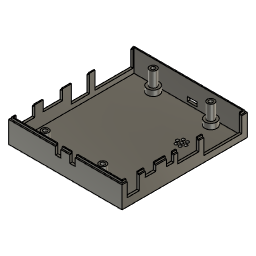
VersaTermTop (Autodesk Fusion 360 design; units mm, degrees)
Autodesk Fusion 360 part; units mm, degrees
(part 1 of 3)
box "BoxPrimitive1" add length 104.5 width 94.5 height 20.6 placed x (0, 1, 0) y (-1, 0, 0) z (0, 0, 1) at (94.5, 0, 0) makes body 1
shell "Shell1" thickness 2 removed faces 1 at (31.5, 34.8333, 20.6) on bodies 1
sketch "Sketch3" plane through (0, 0, 2) normal (0, 0, 1) x (-1, 0, 0)
  line L0 (-92.5, -102.5) -> (-2, -102.5)
  line L1 (-2, -102.5) -> (-2, -2)
  line L2 (-2, -2) -> (-92.5, -2)
  line L3 (-92.5, -2) -> (-92.5, -102.5)
  circle A0 centre (-23.25, -97.25) radius 5
  dimension "d7" = 10
  dimension "d8" = 5.25
  dimension "d9" = 21.25
  measures "d7" diameter of A0
  measures "d8" distance of L0 A0.centre
  measures "d9" distance of L1 A0.centre
extrude "Extrude1" add sketch "Sketch3" along normal blind 4.6 contours A0 bodies 1
sketch "Sketch16" plane through (0, 0, 6.6) normal (0, 0, 1) x (-1, 0, 0)
  circle A0 centre (-23.25, -97.25) radius 5
  circle A1 centre (-23.25, -97.25) radius 3
  dimension "d42" = 6
  constraint concentric A0 A1
  measures "d42" diameter of A1
extrude "Extrude7" add sketch "Sketch16" along normal blind 12.4 contours A1 bodies 1
sketch "Sketch18" plane through (0, 0, 2) normal (0, 0, 1) x (-1, 0, 0)
  circle A0 centre (-23.25, -97.25) radius 5
  line L0 (-92.5, -102.5) -> (-2, -102.5)
  line L1 (-2, -102.5) -> (-2, -2)
  line L2 (-2, -2) -> (-92.5, -2)
  line L3 (-92.5, -2) -> (-92.5, -102.5)
  circle A1 centre (-23.25, -97.25) radius 3.125
  dimension "d49" = 6.25
  constraint concentric A0 A1
  measures "d49" diameter of A1
extrude "Extrude8" cut sketch "Sketch18" against normal blind 3.1 from surface at 1.1 contours A1 bodies 1
sketch "Sketch20" plane through (0, 0, 3.1) normal (0, 0, -1) x (1, 0, 0)
  circle A0 centre (23.25, -97.25) radius 3.125
  circle A1 centre (23.25, -97.25) radius 1.65
  dimension "d56" = 3.3
  constraint concentric A0 A1
  measures "d56" diameter of A1
extrude "Extrude10" cut sketch "Sketch20" against normal blind 17 contours A1 bodies 1
pattern_linear "R-Pattern3" count 2 spacing 90 along (0, -1, 0) count 2 spacing 48 along (1, 0, 0) of "Extrude1", "Extrude7", "Extrude8", "Extrude10"
chamfer "Chamfer2" distance 1 angle 45 4 edges at (94.5, 52.25, 0) (47.25, 0, 0) (47.25, 104.5, 0) (0, 52.25, 0) on bodies 1
sketch "Sketch39" plane through (0, 0, 20.6) normal (0, 0, 1) x (-1, 0, 0)
  line L0 (-92.5, -102.5) -> (-92.5, -2)
  line L1 (-92.5, -2) -> (-2, -2)
  line L2 (-2, -2) -> (-2, -102.5)
  line L3 (-2, -102.5) -> (-92.5, -102.5)
  line L4 (-94.5, -104.5) -> (0, -104.5)
  line L5 (0, -104.5) -> (0, 0)
  line L6 (0, 0) -> (-94.5, 0)
  line L7 (-94.5, 0) -> (-94.5, -104.5)
  line L8 (0, -104.5) -> (-94.5, -104.5)
  line L9 (-94.5, -104.5) -> (-94.5, 0)
  line L10 (-94.5, 0) -> (0, 0)
  line L11 (0, 0) -> (0, -104.5)
  line L12 (-93.4, -1.1) -> (-1.1, -1.1)
  line L13 (-1.1, -1.1) -> (-1.1, -103.4)
  line L14 (-1.1, -103.4) -> (-93.4, -103.4)
  line L15 (-93.4, -103.4) -> (-93.4, -1.1)
  dimension "d89" = 1.1
  constraint horizontal L8
  constraint vertical L9
  constraint horizontal L10
  constraint vertical L11
  constraint coincident L6.end L7.start
  constraint coincident L4.end L5.start
extrude "Extrude15" cut sketch "Sketch39" against normal blind 1.6 contours L4 L5 L6 L7 L8 L9 L10 L11 bodies 1
sketch "Sketch27" plane through (94.5, 0, 0) normal (1, 0, 0) x (0, 1, 0)
  line L0 (104.5, 1) -> (104.5, 19)
  line L1 (0, 19) -> (0, 1)
  line L2 (4.39, 20.6) -> (14.39, 20.6)
  line L3 (14.39, 20.6) -> (14.39, 7.6)
  line L4 (14.39, 7.6) -> (4.39, 7.6)
  line L5 (4.39, 7.6) -> (4.39, 20.6)
  line L6 (0, 1) -> (104.5, 1)
  line L7 (104.5, 19) -> (0, 19)
  line L8 (1.1, 20.6) -> (103.4, 20.6)
  dimension "d69" = 13
  dimension "d70" = 10
  dimension "d79" = 4.39
  constraint horizontal L2
  constraint vertical L3
  constraint horizontal L4
  constraint vertical L5
  constraint collinear L2 L8
  measures "d69" distance of L2 L4
  measures "d70" distance of L3 L5
  measures "d79" distance of L1 L5
extrude "Extrude12" cut sketch "Sketch27" against normal blind 2 contours L2 L3 L5 L7 L8 | L3 L4 L5 L7 bodies 1
sketch "Sketch28" plane through (94.5, 0, 0) normal (1, 0, 0) x (0, 1, 0)
  line L0 (0, 19) -> (0, 1)
  line L1 (104.5, 1) -> (104.5, 19)
  line L2 (19.465, 20.6) -> (28.165, 20.6)
  line L3 (28.165, 20.6) -> (28.165, 14.7)
  line L4 (28.165, 14.7) -> (19.465, 14.7)
  line L5 (19.465, 14.7) -> (19.465, 20.6)
  line L6 (4.39, 7.6) -> (4.39, 19)
  line L7 (14.39, 19) -> (14.39, 7.6)
  line L8 (14.39, 7.6) -> (4.39, 7.6)
  line L9 (0, 1) -> (104.5, 1)
  line L10 (4.39, 19) -> (0, 19)
  line L11 (104.5, 19) -> (14.39, 19)
  line L12 (14.39, 20.6) -> (103.4, 20.6)
  dimension "d75" = 8.7
  dimension "d76" = 5.9
  dimension "d80" = 19.465
  constraint horizontal L2
  constraint vertical L3
  constraint horizontal L4
  constraint vertical L5
  constraint collinear L2 L12
  measures "d75" distance of L3 L5
  measures "d76" distance of L2 L4
  measures "d80" distance of L0 L5
extrude "Extrude13" cut sketch "Sketch28" against normal blind 2 contours L2 L3 L5 L11 L12 | L3 L4 L5 L11 bodies 1
sketch "Sketch41" plane through (0, 0, 0) normal (-1, 0, 0) x (0, -1, 0)
  line L0 (-104.5, 19) -> (-104.5, 1)
  line L1 (0, 1) -> (0, 19)
  line L2 (-65.35, 20.6) -> (-50.35, 20.6)
  line L3 (-50.35, 20.6) -> (-50.35, 5.8)
  line L4 (-50.35, 5.8) -> (-65.35, 5.8)
  line L5 (-65.35, 5.8) -> (-65.35, 20.6)
  line L6 (-104.5, 1) -> (0, 1)
  line L7 (0, 19) -> (-104.5, 19)
  line L8 (-28.165, 20.6) -> (-103.4, 20.6)
  dimension "d97" = 14.8
  dimension "d98" = 15
  dimension "d102" = 39.15
  constraint horizontal L2
  constraint vertical L3
  constraint horizontal L4
  constraint vertical L5
  constraint collinear L2 L8
  measures "d97" distance of L2 L4
  measures "d98" distance of L3 L5
  measures "d102" distance of L0 L5
extrude "Extrude17" cut sketch "Sketch41" against normal blind 2 contours L3 L4 L5 L7 | L2 L3 L5 L7 L8 bodies 1
sketch "Sketch42" plane through (0, 0, 0) normal (-1, 0, 0) x (0, -1, 0)
  line L0 (-65.35, 5.8) -> (-65.35, 19)
  line L1 (-104.5, 19) -> (-104.5, 1)
  line L2 (0, 1) -> (0, 19)
  line L3 (-50.35, 19) -> (-50.35, 5.8)
  line L4 (-50.35, 5.8) -> (-65.35, 5.8)
  line L5 (-42.94, 20.6) -> (-26.94, 20.6)
  line L6 (-26.94, 20.6) -> (-26.94, 12)
  line L7 (-26.94, 12) -> (-42.94, 12)
  line L8 (-42.94, 12) -> (-42.94, 20.6)
  line L9 (-104.5, 1) -> (0, 1)
  line L10 (-65.35, 19) -> (-104.5, 19)
  line L11 (0, 19) -> (-50.35, 19)
  line L12 (-28.165, 20.6) -> (-103.4, 20.6)
  dimension "d103" = 16
  dimension "d104" = 8.6
  dimension "d105" = 26.94
  constraint horizontal L5
  constraint vertical L6
  constraint horizontal L7
  constraint vertical L8
  constraint collinear L5 L12
  measures "d103" distance of L6 L8
  measures "d104" distance of L5 L7
  measures "d105" distance of L2 L6
extrude "Extrude18" cut sketch "Sketch42" against normal blind 2 contours L6 L7 L8 L11 | L5 L6 L8 L11 L12 bodies 1
sketch "Sketch43" plane through (0, 0, 0) normal (-1, 0, 0) x (0, -1, 0)
  line L0 (-42.94, 12) -> (-42.94, 19)
  line L1 (-50.35, 19) -> (-50.35, 5.8)
  line L2 (-50.35, 5.8) -> (-65.35, 5.8)
  line L3 (-65.35, 5.8) -> (-65.35, 19)
  line L4 (-104.5, 19) -> (-104.5, 1)
  line L5 (0, 1) -> (0, 19)
  line L6 (-26.94, 19) -> (-26.94, 12)
  line L7 (-26.94, 12) -> (-42.94, 12)
  line L8 (-19.83, 20.6) -> (-4.33, 20.6)
  line L9 (-4.33, 20.6) -> (-4.33, 11.5)
  line L10 (-4.33, 11.5) -> (-19.83, 11.5)
  line L11 (-19.83, 11.5) -> (-19.83, 20.6)
  line L12 (-104.5, 1) -> (0, 1)
  line L13 (-42.94, 19) -> (-50.35, 19)
  line L14 (-65.35, 19) -> (-104.5, 19)
  line L15 (0, 19) -> (-26.94, 19)
  line L16 (-2, 20.6) -> (-26.94, 20.6)
  dimension "d108" = 4.33
  dimension "d109" = 15.5
  dimension "d110" = 9.1
  constraint horizontal L8
  constraint vertical L9
  constraint horizontal L10
  constraint vertical L11
  constraint collinear L8 L16
  measures "d108" distance of L5 L9
  measures "d109" distance of L9 L11
  measures "d110" distance of L8 L10
extrude "Extrude19" cut sketch "Sketch43" against normal blind 2 contours L9 L10 L11 L15 | L8 L9 L11 L15 L16 bodies 1
sketch "Sketch44" plane through (0, 0, 0) normal (-1, 0, 0) x (0, -1, 0)
  line L0 (-19.83, 11.5) -> (-19.83, 19)
  line L1 (-26.94, 19) -> (-26.94, 12)
  line L2 (-26.94, 12) -> (-42.94, 12)
  line L3 (-42.94, 12) -> (-42.94, 19)
  line L4 (-50.35, 19) -> (-50.35, 5.8)
  line L5 (-50.35, 5.8) -> (-65.35, 5.8)
  line L6 (-65.35, 5.8) -> (-65.35, 19)
  line L7 (-104.5, 19) -> (-104.5, 1)
  line L8 (0, 1) -> (0, 19)
  line L9 (-4.33, 19) -> (-4.33, 11.5)
  line L10 (-4.33, 11.5) -> (-19.83, 11.5)
  line L11 (-101.776, 20.6) -> (-69.966, 20.6)
  line L12 (-69.966, 20.6) -> (-69.966, 6.05)
  line L13 (-69.966, 6.05) -> (-101.776, 6.05)
  line L14 (-101.776, 6.05) -> (-101.776, 20.6)
  line L15 (-104.5, 1) -> (0, 1)
  line L16 (-19.83, 19) -> (-26.94, 19)
  line L17 (-42.94, 19) -> (-50.35, 19)
  line L18 (-65.35, 19) -> (-104.5, 19)
  line L19 (0, 19) -> (-4.33, 19)
  line L20 (-28.165, 20.6) -> (-103.4, 20.6)
  dimension "d113" = 31.81
  dimension "d114" = 14.55
  dimension "d115" = 2.724
  constraint horizontal L11
  constraint vertical L12
  constraint horizontal L13
  constraint vertical L14
  constraint collinear L11 L20
  measures "d113" distance of L12 L14
  measures "d114" distance of L11 L13
  measures "d115" distance of L7 L14
extrude "Extrude20" cut sketch "Sketch44" against normal blind 2 contours L12 L13 L14 L18 | L11 L12 L14 L18 L20 bodies 1
sketch "Sketch45" plane through (94.5, 0, 0) normal (1, 0, 0) x (0, 1, 0)
  line L0 (46.5, 20.6) -> (64, 20.6)
  line L1 (64, 20.6) -> (64, 10.9)
  line L2 (64, 10.9) -> (46.5, 10.9)
  line L3 (46.5, 10.9) -> (46.5, 20.6)
  line L4 (104.5, 1) -> (104.5, 18.5)
  line L5 (19.465, 14.7) -> (19.465, 19)
  line L6 (14.39, 19) -> (14.39, 7.6)
  line L7 (14.39, 7.6) -> (4.39, 7.6)
  line L8 (4.39, 7.6) -> (4.39, 19)
  line L9 (0, 19) -> (0, 1)
  line L10 (0, 1) -> (104.5, 1)
  line L11 (104.5, 1) -> (104.5, 19)
  line L12 (28.165, 19) -> (28.165, 14.7)
  line L13 (28.165, 14.7) -> (19.465, 14.7)
  line L14 (19.465, 19) -> (14.39, 19)
  line L15 (4.39, 19) -> (0, 19)
  line L16 (104.5, 19) -> (28.165, 19)
  line L17 (28.165, 20.6) -> (103.4, 20.6)
  dimension "d118" = 40.5
  dimension "d119" = 17.5
  dimension "d120" = 9.7
  constraint horizontal L0
  constraint vertical L1
  constraint horizontal L2
  constraint vertical L3
  constraint collinear L0 L17
  measures "d118" distance of L1 L4
  measures "d119" distance of L1 L3
  measures "d120" distance of L0 L2
extrude "Extrude21" cut sketch "Sketch45" against normal blind 2 contours L0 L1 L3 L16 L17 | L1 L2 L3 L16 bodies 1
sketch "Sketch46" plane through (94.5, 0, 0) normal (1, 0, 0) x (0, 1, 0)
  line L0 (46.5, 10.9) -> (46.5, 19)
  line L1 (28.165, 19) -> (28.165, 14.7)
  line L2 (28.165, 14.7) -> (19.465, 14.7)
  line L3 (19.465, 14.7) -> (19.465, 19)
  line L4 (14.39, 19) -> (14.39, 7.6)
  line L5 (14.39, 7.6) -> (4.39, 7.6)
  line L6 (4.39, 7.6) -> (4.39, 19)
  line L7 (0, 19) -> (0, 1)
  line L8 (0, 1) -> (104.5, 1)
  line L9 (104.5, 1) -> (104.5, 19)
  line L10 (64, 19) -> (64, 10.9)
  line L11 (64, 10.9) -> (46.5, 10.9)
  line L12 (68.186, 20.6) -> (99.746, 20.6)
  line L13 (99.746, 20.6) -> (99.746, 6.05)
  line L14 (99.746, 6.05) -> (68.186, 6.05)
  line L15 (68.186, 6.05) -> (68.186, 20.6)
  line L16 (46.5, 19) -> (28.165, 19)
  line L17 (19.465, 19) -> (14.39, 19)
  line L18 (4.39, 19) -> (0, 19)
  line L19 (104.5, 19) -> (64, 19)
  line L20 (64, 20.6) -> (103.4, 20.6)
  dimension "d124" = 4.754
  dimension "d125" = 31.56
  dimension "d126" = 14.55
  constraint horizontal L12
  constraint vertical L13
  constraint horizontal L14
  constraint vertical L15
  constraint collinear L12 L20
  measures "d124" distance of L9 L13
  measures "d125" distance of L13 L15
  measures "d126" distance of L12 L14
extrude "Extrude22" cut sketch "Sketch46" against normal blind 2 contours L13 L14 L15 L19 | L12 L13 L15 L19 L20 bodies 1
sketch "Sketch47" plane through (94.5, 0, 0) normal (1, 0, 0) x (0, 1, 0)
  line L0 (68.186, 6.05) -> (68.186, 19)
  line L1 (64, 19) -> (64, 10.9)
  line L2 (64, 10.9) -> (46.5, 10.9)
  line L3 (46.5, 10.9) -> (46.5, 19)
  line L4 (28.165, 19) -> (28.165, 14.7)
  line L5 (28.165, 14.7) -> (19.465, 14.7)
  line L6 (19.465, 14.7) -> (19.465, 19)
  line L7 (14.39, 19) -> (14.39, 7.6)
  line L8 (14.39, 7.6) -> (4.39, 7.6)
  line L9 (4.39, 7.6) -> (4.39, 19)
  line L10 (0, 19) -> (0, 1)
  line L11 (0, 1) -> (104.5, 1)
  line L12 (104.5, 1) -> (104.5, 19)
  line L13 (99.746, 19) -> (99.746, 6.05)
  line L14 (99.746, 6.05) -> (68.186, 6.05)
  line L15 (37.12, 20.6) -> (43.12, 20.6)
  line L16 (43.12, 20.6) -> (43.12, 13.6)
  line L17 (43.12, 13.6) -> (37.12, 13.6)
  line L18 (37.12, 13.6) -> (37.12, 20.6)
  line L19 (68.186, 19) -> (64, 19)
  line L20 (46.5, 19) -> (28.165, 19)
  line L21 (19.465, 19) -> (14.39, 19)
  line L22 (4.39, 19) -> (0, 19)
  line L23 (104.5, 19) -> (99.746, 19)
  line L24 (28.165, 20.6) -> (46.5, 20.6)
  dimension "d129" = 6
  dimension "d130" = 7
  dimension "d131" = 37.12
  constraint horizontal L15
  constraint vertical L16
  constraint horizontal L17
  constraint vertical L18
  constraint collinear L15 L24
  measures "d129" distance of L16 L18
  measures "d130" distance of L15 L17
  measures "d131" distance of L10 L18
extrude "Extrude23" cut sketch "Sketch47" against normal blind 2 contours L15 L16 L18 L20 L24 | L16 L17 L18 L20 bodies 1
sketch "Sketch48" plane through (0, 0, 2) normal (0, 0, 1) x (-1, 0, 0)
  circle A0 centre (-71.25, -7.25) radius 5
  circle A1 centre (-71.25, -97.25) radius 5
  circle A2 centre (-23.25, -7.25) radius 5
  circle A3 centre (-23.25, -97.25) radius 5
  line L0 (-92.5, -102.5) -> (-2, -102.5)
  line L1 (-2, -102.5) -> (-2, -2)
  line L2 (-2, -2) -> (-92.5, -2)
  line L3 (-92.5, -2) -> (-92.5, -102.5)
  circle A4 centre (-73.37, -14.47) radius 3.5
  dimension "d134" = 19.13
  dimension "d135" = 7
  dimension "d136" = 12.47
  measures "d134" distance of L3 A4.centre
  measures "d135" diameter of A4
  measures "d136" distance of L2 A4.centre
sketch "Sketch49" plane through (0, 0, 0) normal (0, -1, 0) x (1, 0, 0)
  line L0 (0, 1) -> (94.5, 1)
  line L1 (94.5, 1) -> (94.5, 19)
  line L2 (0, 19) -> (0, 1)
  line L3 (51, 20.6) -> (55.5, 20.6)
  line L4 (55.5, 20.6) -> (55.5, 12.8)
  line L5 (55.5, 12.8) -> (51, 12.8)
  line L6 (51, 12.8) -> (51, 20.6)
  line L7 (94.5, 19) -> (0, 19)
  line L8 (1.1, 20.6) -> (93.4, 20.6)
  dimension "d137" = 39
  dimension "d138" = 4.5
  dimension "d139" = 7.8
  constraint horizontal L3
  constraint vertical L4
  constraint horizontal L5
  constraint vertical L6
  constraint collinear L3 L8
  measures "d137" distance of L1 L4
  measures "d138" distance of L4 L6
  measures "d139" distance of L3 L5
extrude "Extrude24" cut sketch "Sketch49" against normal blind 2 contours L4 L5 L6 L7 | L3 L4 L6 L7 L8 bodies 1
sketch "Sketch50" plane through (0, 0, 0) normal (0, -1, 0) x (1, 0, 0)
  line L0 (51, 12.8) -> (51, 19)
  line L1 (0, 19) -> (0, 1)
  line L2 (0, 1) -> (94.5, 1)
  line L3 (94.5, 1) -> (94.5, 19)
  line L4 (55.5, 19) -> (55.5, 12.8)
  line L5 (55.5, 12.8) -> (51, 12.8)
  line L6 (39, 20.6) -> (43.5, 20.6)
  line L7 (43.5, 20.6) -> (43.5, 12.8)
  line L8 (43.5, 12.8) -> (39, 12.8)
  line L9 (39, 12.8) -> (39, 20.6)
  line L10 (51, 19) -> (0, 19)
  line L11 (94.5, 19) -> (55.5, 19)
  line L12 (1.1, 20.6) -> (51, 20.6)
  dimension "d142" = 51
  dimension "d143" = 4.5
  dimension "d144" = 7.8
  constraint horizontal L6
  constraint vertical L7
  constraint horizontal L8
  constraint vertical L9
  constraint collinear L6 L12
  measures "d142" distance of L3 L7
  measures "d143" distance of L7 L9
  measures "d144" distance of L6 L8
extrude "Extrude25" cut sketch "Sketch50" against normal blind 2 contours L6 L7 L9 L10 L12 | L7 L8 L9 L10 bodies 1
extrude "Extrude26" add sketch "Sketch48" along normal blind 6 separate body contours A0 A4 | A0 A4 picked at (-72.1915, -11.8436) picked at (-71.939, -13.8039) makes body 2
combine "Combine1" operation cut target body 1 tool bodies 2
sketch "Sketch57" plane through (0, 0, 2) normal (0, 0, 1) x (-1, 0, 0)
  arc A0 (-70.6903, -12.2186) -> (-74.4071, -11.1272) centre (-71.25, -7.25) ccw
  arc A1 (-70.6903, -12.2186) -> (-74.4071, -11.1272) centre (-73.37, -14.47) ccw
  circle A2 centre (-71.25, -97.25) radius 5
  circle A3 centre (-23.25, -7.25) radius 5
  circle A4 centre (-23.25, -97.25) radius 5
  line L0 (-92.5, -102.5) -> (-2, -102.5)
  line L1 (-2, -102.5) -> (-2, -2)
  line L2 (-2, -2) -> (-92.5, -2)
  line L3 (-92.5, -2) -> (-92.5, -102.5)
  circle A5 centre (-72.05, -72.25) radius 1.25
  dimension "d149" = 2.5
  dimension "d150" = 30.25
  dimension "d151" = 20.45
  measures "d149" diameter of A5
  measures "d150" distance of L0 A5.centre
  measures "d151" distance of L3 A5.centre
extrude "Extrude27" cut sketch "Sketch57" against normal blind 2 contours A5 bodies 1
sketch "Sketch58" plane through (0, 0, 2) normal (0, 0, 1) x (-1, 0, 0)
  circle A0 centre (-72.05, -72.25) radius 1.25
  arc A1 (-70.6903, -12.2186) -> (-74.4071, -11.1272) centre (-71.25, -7.25) ccw
  arc A2 (-70.6903, -12.2186) -> (-74.4071, -11.1272) centre (-73.37, -14.47) ccw
  circle A3 centre (-71.25, -97.25) radius 5
  circle A4 centre (-23.25, -7.25) radius 5
  circle A5 centre (-23.25, -97.25) radius 5
  line L0 (-92.5, -102.5) -> (-2, -102.5)
  line L1 (-2, -102.5) -> (-2, -2)
  line L2 (-2, -2) -> (-92.5, -2)
  line L3 (-92.5, -2) -> (-92.5, -102.5)
  circle A6 centre (-68.55, -72.25) radius 1.25
  dimension "d154" = 23.95
  dimension "d155" = 30.25
  dimension "d158" = 2.5
  measures "d154" distance of L3 A6.centre
  measures "d155" distance of L0 A6.centre
  measures "d158" diameter of A6
extrude "Extrude28" cut sketch "Sketch58" against normal blind 2 contours A6 bodies 1
pattern_circular "C-Pattern1" count 6 over 360 about axis through (72.05, 72.25, 2) along (0, 0, -1) of 1 faces at (68.1519, 71.0651, 0.6667) on bodies 1
sketch "Sketch61" plane through (0, 0, 2) normal (0, 0, 1) x (1, 0, 0)
  circle A0 centre (72.05, 65.25) radius 1.25
  line L0 (92.5, 68.186) -> (92.5, 100.246)
  line L1 (2, 102.5) -> (92.5, 102.5)
  dimension "d163" = 20.45
  dimension "d164" = 2.5
  dimension "d165" = 37.25
  measures "d163" distance of A0.centre L0
  measures "d164" diameter of A0
  measures "d165" distance of A0.centre L1
extrude "Extrude29" [suppressed]
pattern_circular "C-Pattern2" [suppressed]
sketch "Sketch62" plane through (0, 104.5, 0) normal (0, 1, 0) x (-1, 0, 0)
  line L0 (0, 19) -> (-94.5, 19)
  line L1 (-94.5, 19) -> (-94.5, 1)
  line L2 (-94.5, 1) -> (0, 1)
  line L3 (0, 1) -> (0, 19)
  line L4 (-54.5, 7.5) -> (-46.5, 7.5)
  line L5 (-46.5, 7.5) -> (-46.5, 4)
  line L6 (-46.5, 4) -> (-54.5, 4)
  line L7 (-54.5, 4) -> (-54.5, 7.5)
  dimension "d171" = 11.5
  dimension "d172" = 8
  dimension "d173" = 3.5
  dimension "d206" = 40
  constraint horizontal L4
  constraint vertical L5
  constraint horizontal L6
  constraint vertical L7
  measures "d171" distance of L0 L4
  measures "d172" distance of L5 L7
  measures "d173" distance of L4 L6
  measures "d206" distance of L1 L4.start
extrude "Extrude30" cut sketch "Sketch62" against normal blind 2 contours L4 L5 L6 L7 bodies 1
sketch "Sketch63" plane through (94.5, 0, 0) normal (1, 0, 0) x (0, 1, 0)
  line L0 (43.12, 19) -> (43.12, 13.6)
  line L1 (43.12, 13.6) -> (37.12, 13.6)
  line L2 (37.12, 13.6) -> (37.12, 19)
  line L3 (37.12, 19) -> (28.165, 19)
  line L4 (28.165, 19) -> (28.165, 14.7)
  line L5 (28.165, 14.7) -> (19.465, 14.7)
  line L6 (19.465, 14.7) -> (19.465, 19)
  line L7 (19.465, 19) -> (14.39, 19)
  line L8 (14.39, 19) -> (14.39, 7.6)
  line L9 (14.39, 7.6) -> (4.39, 7.6)
  line L10 (4.39, 7.6) -> (4.39, 19)
  line L11 (4.39, 19) -> (0, 19)
  line L12 (0, 19) -> (0, 1)
  line L13 (0, 1) -> (104.5, 1)
  line L14 (104.5, 1) -> (104.5, 19)
  line L15 (104.5, 19) -> (99.746, 19)
  line L16 (99.746, 19) -> (99.746, 6.05)
  line L17 (99.746, 6.05) -> (68.186, 6.05)
  line L18 (68.186, 6.05) -> (68.186, 19)
  line L19 (68.186, 19) -> (64, 19)
  line L20 (64, 19) -> (64, 10.9)
  line L21 (64, 10.9) -> (46.5, 10.9)
  line L22 (46.5, 10.9) -> (46.5, 19)
  line L23 (46.5, 19) -> (43.12, 19)
  line L24 (68.186, 6.05) -> (99.746, 6.05)
  line L25 (99.746, 6.05) -> (99.746, 1)
  line L26 (99.746, 1) -> (68.186, 1)
  line L27 (68.186, 1) -> (68.186, 6.05)
  constraint horizontal L24
  constraint vertical L25
  constraint horizontal L26
  constraint vertical L27
  constraint coincident L13 L25.end
  constraint coincident L17.end L18.start
  constraint collinear L16 L25
sketch "Sketch71" plane through (0, 0, 0) normal (0, 0, -1) x (1, 0, 0)
  circle A0 centre (70.3, -69.2189) radius 1.25
  circle A1 centre (73.8, -69.2189) radius 1.25
  circle A2 centre (75.55, -72.25) radius 1.25
  circle A3 centre (73.8, -75.2811) radius 1.25
  circle A4 centre (70.3, -75.2811) radius 1.25
  circle A5 centre (68.55, -72.25) radius 1.25
  circle A6 centre (72.05, -72.25) radius 1.25
  circle A7 centre (23.25, -97.25) radius 3.125
  circle A8 centre (23.25, -7.25) radius 3.125
  circle A9 centre (71.25, -97.25) radius 3.125
  circle A10 centre (71.25, -7.25) radius 3.125
  line L0 (1, -1) -> (1, -103.5)
  line L1 (1, -103.5) -> (93.5, -103.5)
  line L2 (93.5, -103.5) -> (93.5, -1)
  line L3 (93.5, -1) -> (1, -1)
  line L4 (84.5763, -29.4929) -> (85.1763, -29.4929)
  line L5 (85.1763, -29.4929) -> (85.1763, -4.4181)
  line L6 (85.1763, -4.4181) -> (84.5763, -4.4181)
  line L7 (84.5763, -4.4181) -> (84.5763, -29.4929)
  line L8 (8.4823, -82.4804) -> (8.4823, -83.5039)
  line L9 (8.4823, -83.5039) -> (3.7019, -81.8788)
  line L10 (3.7019, -81.8788) -> (3.7019, -80.7736)
  line L11 (3.7019, -80.7736) -> (8.4823, -79.1518)
  line L12 (8.4823, -79.1518) -> (8.4823, -80.1752)
  line L13 (8.4823, -80.1752) -> (5.6376, -81.0744)
  spline S0 degree 2 poles (5.6376, -81.0744) (5.3859, -81.1496) (5.0507, -81.2297) knots 0 0 0 1 1 1
  spline S1 degree 2 poles (5.0507, -81.2297) (4.7156, -81.3098) (4.5848, -81.3295) knots 0 0 0 1 1 1
  spline S2 degree 2 poles (4.5848, -81.3295) (4.8856, -81.3654) (5.6376, -81.5747) knots 0 0 0 1 1 1
  line L14 (5.6376, -81.5747) -> (8.4823, -82.4804)
  line L15 (6.3864, -85.9202) -> (6.3864, -87.8167)
  line L16 (6.3864, -87.8167) -> (3.9079, -87.8167)
  spline S3 degree 2 poles (3.9079, -87.8167) (3.7575, -87.3556) (3.697, -86.9485) knots 0 0 0 1 1 1
  spline S4 degree 2 poles (3.697, -86.9485) (3.6365, -86.5415) (3.6365, -86.1164) knots 0 0 0 1 1 1
  spline S5 degree 2 poles (3.6365, -86.1164) (3.6365, -85.0341) (4.2725, -84.4635) knots 0 0 0 1 1 1
  spline S6 degree 2 poles (4.2725, -84.4635) (4.9085, -83.893) (6.0987, -83.893) knots 0 0 0 1 1 1
  spline S7 degree 2 poles (6.0987, -83.893) (7.2562, -83.893) (7.9036, -84.5551) knots 0 0 0 1 1 1
  spline S8 degree 2 poles (7.9036, -84.5551) (8.551, -85.2172) (8.551, -86.391) knots 0 0 0 1 1 1
  spline S9 degree 2 poles (8.551, -86.391) (8.551, -87.1267) (8.2567, -87.8101) knots 0 0 0 1 1 1
  line L17 (8.2567, -87.8101) -> (7.4458, -87.4733)
  spline S10 degree 2 poles (7.4458, -87.4733) (7.7074, -86.9502) (7.7074, -86.3845) knots 0 0 0 1 1 1
  spline S11 degree 2 poles (7.7074, -86.3845) (7.7074, -85.7273) (7.266, -85.3316) knots 0 0 0 1 1 1
  spline S12 degree 2 poles (7.266, -85.3316) (6.8246, -84.936) (6.079, -84.936) knots 0 0 0 1 1 1
  spline S13 degree 2 poles (6.079, -84.936) (5.3008, -84.936) (4.8905, -85.2548) knots 0 0 0 1 1 1
  spline S14 degree 2 poles (4.8905, -85.2548) (4.4801, -85.5736) (4.4801, -86.1818) knots 0 0 0 1 1 1
  spline S15 degree 2 poles (4.4801, -86.1818) (4.4801, -86.4989) (4.5455, -86.8259) knots 0 0 0 1 1 1
  line L18 (4.5455, -86.8259) -> (5.5428, -86.8259)
  line L19 (5.5428, -86.8259) -> (5.5428, -85.9202)
  line L20 (5.5428, -85.9202) -> (6.3864, -85.9202)
  line L21 (3.7019, -91.881) -> (4.8398, -91.5344)
  line L22 (4.8398, -91.5344) -> (4.8398, -89.7916)
  line L23 (4.8398, -89.7916) -> (3.7019, -89.445)
  line L24 (3.7019, -89.445) -> (3.7019, -88.3529)
  line L25 (3.7019, -88.3529) -> (8.5019, -90.0401)
  line L26 (8.5019, -90.0401) -> (8.5019, -91.2793)
  line L27 (8.5019, -91.2793) -> (3.7019, -92.9731)
  line L28 (3.7019, -92.9731) -> (3.7019, -91.881)
  spline S16 degree 2 poles (5.6899, -91.2924) (7.2365, -90.8118) (7.4393, -90.7513) knots 0 0 0 1 1 1
  spline S17 degree 2 poles (7.4393, -90.7513) (7.642, -90.6908) (7.7597, -90.6646) knots 0 0 0 1 1 1
  spline S18 degree 2 poles (7.7597, -90.6646) (7.3412, -90.5567) (5.6899, -90.0466) knots 0 0 0 1 1 1
  line L29 (5.6899, -90.0466) -> (5.6899, -91.2924)
  line L30 (6.0694, -51.955) -> (6.0694, -52.2885)
  spline S19 degree 2 poles (6.0694, -52.2885) (6.0694, -52.756) (6.2541, -52.9882) knots 0 0 0 1 1 1
  spline S20 degree 2 poles (6.2541, -52.9882) (6.4389, -53.2204) (6.792, -53.2204) knots 0 0 0 1 1 1
  spline S21 degree 2 poles (6.792, -53.2204) (7.1484, -53.2204) (7.3184, -53.0258) knots 0 0 0 1 1 1
  spline S22 degree 2 poles (7.3184, -53.0258) (7.4884, -52.8313) (7.4884, -52.416) knots 0 0 0 1 1 1
  line L31 (7.4884, -52.416) -> (7.4884, -51.955)
  line L32 (7.4884, -51.955) -> (6.0694, -51.955)
  spline S23 degree 2 poles (6.828, -54.2438) (6.0563, -54.2438) (5.6476, -53.7615) knots 0 0 0 1 1 1
  spline S24 degree 2 poles (5.6476, -53.7615) (5.2389, -53.2792) (5.2389, -52.3898) knots 0 0 0 1 1 1
  line L33 (5.2389, -52.3898) -> (5.2389, -51.955)
  line L34 (5.2389, -51.955) -> (3.5386, -51.955)
  line L35 (3.5386, -51.955) -> (3.5386, -50.9413)
  line L36 (3.5386, -50.9413) -> (8.319, -50.9413)
  line L37 (8.319, -50.9413) -> (8.319, -52.4683)
  spline S25 degree 2 poles (8.319, -52.4683) (8.319, -53.3381) (7.9446, -53.7909) knots 0 0 0 1 1 1
  spline S26 degree 2 poles (7.9446, -53.7909) (7.5702, -54.2438) (6.828, -54.2438) knots 0 0 0 1 1 1
  spline S27 degree 2 poles (4.8661, -57.968) (4.2187, -57.968) (3.8459, -57.5021) knots 0 0 0 1 1 1
  spline S28 degree 2 poles (3.8459, -57.5021) (3.4732, -57.0362) (3.4732, -56.2056) knots 0 0 0 1 1 1
  spline S29 degree 2 poles (3.4732, -56.2056) (3.4732, -55.4405) (3.7609, -54.852) knots 0 0 0 1 1 1
  line L38 (3.7609, -54.852) -> (4.7026, -54.852)
  spline S30 degree 2 poles (4.7026, -54.852) (4.4868, -55.3359) (4.3985, -55.671) knots 0 0 0 1 1 1
  spline S31 degree 2 poles (4.3985, -55.671) (4.3102, -56.0062) (4.3102, -56.2841) knots 0 0 0 1 1 1
  spline S32 degree 2 poles (4.3102, -56.2841) (4.3102, -56.6176) (4.4378, -56.7958) knots 0 0 0 1 1 1
  spline S33 degree 2 poles (4.4378, -56.7958) (4.5653, -56.974) (4.8171, -56.974) knots 0 0 0 1 1 1
  spline S34 degree 2 poles (4.8171, -56.974) (4.9577, -56.974) (5.0672, -56.8956) knots 0 0 0 1 1 1
  spline S35 degree 2 poles (5.0672, -56.8956) (5.1767, -56.8171) (5.2781, -56.665) knots 0 0 0 1 1 1
  spline S36 degree 2 poles (5.2781, -56.665) (5.3795, -56.513) (5.6018, -56.0454) knots 0 0 0 1 1 1
  spline S37 degree 2 poles (5.6018, -56.0454) (5.8078, -55.6073) (5.9974, -55.3882) knots 0 0 0 1 1 1
  spline S38 degree 2 poles (5.9974, -55.3882) (6.1871, -55.1691) (6.4389, -55.0383) knots 0 0 0 1 1 1
  spline S39 degree 2 poles (6.4389, -55.0383) (6.6906, -54.9075) (7.0274, -54.9075) knots 0 0 0 1 1 1
  spline S40 degree 2 poles (7.0274, -54.9075) (7.6617, -54.9075) (8.0247, -55.3375) knots 0 0 0 1 1 1
  spline S41 degree 2 poles (8.0247, -55.3375) (8.3876, -55.7675) (8.3876, -56.5261) knots 0 0 0 1 1 1
  spline S42 degree 2 poles (8.3876, -56.5261) (8.3876, -56.8988) (8.2993, -57.2372) knots 0 0 0 1 1 1
  spline S43 degree 2 poles (8.2993, -57.2372) (8.2111, -57.5757) (8.0508, -57.9451) knots 0 0 0 1 1 1
  line L39 (8.0508, -57.9451) -> (7.2628, -57.6182)
  spline S44 degree 2 poles (7.2628, -57.6182) (7.4198, -57.2356) (7.4819, -56.9855) knots 0 0 0 1 1 1
  spline S45 degree 2 poles (7.4819, -56.9855) (7.544, -56.7353) (7.544, -56.4934) knots 0 0 0 1 1 1
  spline S46 degree 2 poles (7.544, -56.4934) (7.544, -56.2056) (7.41, -56.052) knots 0 0 0 1 1 1
  spline S47 degree 2 poles (7.41, -56.052) (7.2759, -55.8983) (7.0601, -55.8983) knots 0 0 0 1 1 1
  spline S48 degree 2 poles (7.0601, -55.8983) (6.926, -55.8983) (6.8263, -55.9604) knots 0 0 0 1 1 1
  spline S49 degree 2 poles (6.8263, -55.9604) (6.7266, -56.0225) (6.6334, -56.1582) knots 0 0 0 1 1 1
  spline S50 degree 2 poles (6.6334, -56.1582) (6.5402, -56.2939) (6.2983, -56.8007) knots 0 0 0 1 1 1
  spline S51 degree 2 poles (6.2983, -56.8007) (5.9778, -57.471) (5.6557, -57.7195) knots 0 0 0 1 1 1
  spline S52 degree 2 poles (5.6557, -57.7195) (5.3337, -57.968) (4.8661, -57.968) knots 0 0 0 1 1 1
  line L40 (8.319, -60.9664) -> (3.5386, -59.1844)
  line L41 (3.5386, -59.1844) -> (3.5386, -58.2787)
  line L42 (3.5386, -58.2787) -> (8.319, -60.0607)
  line L43 (8.319, -60.0607) -> (8.319, -60.9664)
  line L44 (3.5386, -64.6089) -> (3.5386, -61.2672)
  line L45 (3.5386, -61.2672) -> (4.2416, -61.2672)
  line L46 (4.2416, -61.2672) -> (5.4547, -62.4672)
  spline S53 degree 2 poles (5.4547, -62.4672) (6.0007, -63.0002) (6.2116, -63.1637) knots 0 0 0 1 1 1
  spline S54 degree 2 poles (6.2116, -63.1637) (6.4225, -63.3272) (6.6023, -63.3991) knots 0 0 0 1 1 1
  spline S55 degree 2 poles (6.6023, -63.3991) (6.7822, -63.471) (6.9751, -63.471) knots 0 0 0 1 1 1
  spline S56 degree 2 poles (6.9751, -63.471) (7.2628, -63.471) (7.4034, -63.3125) knots 0 0 0 1 1 1
  spline S57 degree 2 poles (7.4034, -63.3125) (7.544, -63.1539) (7.544, -62.889) knots 0 0 0 1 1 1
  spline S58 degree 2 poles (7.544, -62.889) (7.544, -62.6111) (7.4165, -62.3495) knots 0 0 0 1 1 1
  spline S59 degree 2 poles (7.4165, -62.3495) (7.289, -62.0879) (7.0536, -61.8035) knots 0 0 0 1 1 1
  line L47 (7.0536, -61.8035) -> (7.7042, -61.2541)
  spline S60 degree 2 poles (7.7042, -61.2541) (8.0051, -61.6073) (8.1293, -61.8394) knots 0 0 0 1 1 1
  spline S61 degree 2 poles (8.1293, -61.8394) (8.2536, -62.0716) (8.3206, -62.3462) knots 0 0 0 1 1 1
  spline S62 degree 2 poles (8.3206, -62.3462) (8.3876, -62.6209) (8.3876, -62.961) knots 0 0 0 1 1 1
  spline S63 degree 2 poles (8.3876, -62.961) (8.3876, -63.4089) (8.2241, -63.7522) knots 0 0 0 1 1 1
  spline S64 degree 2 poles (8.2241, -63.7522) (8.0607, -64.0956) (7.7664, -64.2852) knots 0 0 0 1 1 1
  spline S65 degree 2 poles (7.7664, -64.2852) (7.4721, -64.4748) (7.0928, -64.4748) knots 0 0 0 1 1 1
  spline S66 degree 2 poles (7.0928, -64.4748) (6.7626, -64.4748) (6.4732, -64.3588) knots 0 0 0 1 1 1
  spline S67 degree 2 poles (6.4732, -64.3588) (6.1838, -64.2427) (5.8797, -63.9991) knots 0 0 0 1 1 1
  spline S68 degree 2 poles (5.8797, -63.9991) (5.5756, -63.7555) (5.0132, -63.1408) knots 0 0 0 1 1 1
  line L48 (5.0132, -63.1408) -> (4.4345, -62.5261)
  line L49 (4.4345, -62.5261) -> (4.3887, -62.5261)
  line L50 (4.3887, -62.5261) -> (4.3887, -64.6089)
  line L51 (4.3887, -64.6089) -> (3.5386, -64.6089)
  line L52 (3.5013, -30.0411) -> (3.5027, -29.0307)
  line L53 (3.5027, -29.0307) -> (5.5659, -29.0336)
  line L54 (5.5659, -29.0336) -> (5.5686, -27.1405)
  line L55 (5.5686, -27.1405) -> (3.5054, -27.1375)
  line L56 (3.5054, -27.1375) -> (3.5068, -26.1239)
  line L57 (3.5068, -26.1239) -> (8.2872, -26.1307)
  line L58 (8.2872, -26.1307) -> (8.2858, -27.1443)
  line L59 (8.2858, -27.1443) -> (6.4122, -27.1417)
  line L60 (6.4122, -27.1417) -> (6.4095, -29.0348)
  line L61 (6.4095, -29.0348) -> (8.2831, -29.0375)
  line L62 (8.2831, -29.0375) -> (8.2816, -30.0479)
  line L63 (8.2816, -30.0479) -> (3.5013, -30.0411)
  spline S69 degree 2 poles (5.9299, -35.2173) (4.7495, -35.2156) (4.1226, -34.5428) knots 0 0 0 1 1 1
  spline S70 degree 2 poles (4.1226, -34.5428) (3.4958, -33.8699) (3.4976, -32.6013) knots 0 0 0 1 1 1
  line L64 (3.4976, -32.6013) -> (3.4995, -31.2476)
  line L65 (3.4995, -31.2476) -> (8.2799, -31.2544)
  line L66 (8.2799, -31.2544) -> (8.2778, -32.7552)
  spline S71 degree 2 poles (8.2778, -32.7552) (8.2761, -33.9258) (7.6572, -34.5723) knots 0 0 0 1 1 1
  spline S72 degree 2 poles (7.6572, -34.5723) (7.0383, -35.2189) (5.9299, -35.2173) knots 0 0 0 1 1 1
  spline S73 degree 2 poles (5.9052, -34.1644) (7.4452, -34.1666) (7.4472, -32.8064) knots 0 0 0 1 1 1
  line L67 (7.4472, -32.8064) -> (7.4479, -32.2668)
  line L68 (7.4479, -32.2668) -> (4.3351, -32.2624)
  line L69 (4.3351, -32.2624) -> (4.3345, -32.6973)
  spline S74 degree 2 poles (4.3345, -32.6973) (4.3324, -34.1621) (5.9052, -34.1644) knots 0 0 0 1 1 1
  line L70 (3.4896, -38.2285) -> (7.2416, -37.0829)
  line L71 (7.2416, -37.0829) -> (7.2417, -37.0535)
  spline S75 degree 2 poles (7.2417, -37.0535) (6.0972, -37.114) (5.7146, -37.1134) knots 0 0 0 1 1 1
  line L72 (5.7146, -37.1134) -> (3.4912, -37.1103)
  line L73 (3.4912, -37.1103) -> (3.4925, -36.2045)
  line L74 (3.4925, -36.2045) -> (8.2729, -36.2113)
  line L75 (8.2729, -36.2113) -> (8.2709, -37.5912)
  line L76 (8.2709, -37.5912) -> (4.6137, -38.7173)
  line L77 (4.6137, -38.7173) -> (4.6137, -38.7369)
  line L78 (4.6137, -38.7369) -> (8.2675, -39.9421)
  line L79 (8.2675, -39.9421) -> (8.2656, -41.322)
  line L80 (8.2656, -41.322) -> (3.4852, -41.3152)
  line L81 (3.4852, -41.3152) -> (3.4865, -40.3702)
  line L82 (3.4865, -40.3702) -> (5.7492, -40.3734)
  spline S76 degree 2 poles (5.7492, -40.3734) (5.9094, -40.3737) (6.1187, -40.3789) knots 0 0 0 1 1 1
  spline S77 degree 2 poles (6.1187, -40.3789) (6.3279, -40.3841) (7.2303, -40.4246) knots 0 0 0 1 1 1
  line L83 (7.2303, -40.4246) -> (7.2304, -40.3952)
  line L84 (7.2304, -40.3952) -> (3.4883, -39.1571)
  line L85 (3.4883, -39.1571) -> (3.4896, -38.2285)
  line L86 (3.4835, -42.5184) -> (8.2639, -42.5252)
  line L87 (8.2639, -42.5252) -> (8.2624, -43.5389)
  line L88 (8.2624, -43.5389) -> (3.482, -43.5321)
  line L89 (3.482, -43.5321) -> (3.4835, -42.5184)
  line L90 (8.3012, -9.735) -> (5.208, -9.735)
  spline S78 degree 2 poles (5.208, -9.735) (4.6783, -9.735) (4.2794, -9.4979) knots 0 0 0 1 1 1
  spline S79 degree 2 poles (4.2794, -9.4979) (3.8805, -9.2609) (3.668, -8.8129) knots 0 0 0 1 1 1
  spline S80 degree 2 poles (3.668, -8.8129) (3.4555, -8.365) (3.4555, -7.7535) knots 0 0 0 1 1 1
  spline S81 degree 2 poles (3.4555, -7.7535) (3.4555, -6.8315) (3.9279, -6.3214) knots 0 0 0 1 1 1
  spline S82 degree 2 poles (3.9279, -6.3214) (4.4004, -5.8113) (5.2211, -5.8113) knots 0 0 0 1 1 1
  line L91 (5.2211, -5.8113) -> (8.3012, -5.8113)
  line L92 (8.3012, -5.8113) -> (8.3012, -6.8216)
  line L93 (8.3012, -6.8216) -> (5.3748, -6.8216)
  spline S83 degree 2 poles (5.3748, -6.8216) (4.8222, -6.8216) (4.5639, -7.044) knots 0 0 0 1 1 1
  spline S84 degree 2 poles (4.5639, -7.044) (4.3056, -7.2663) (4.3056, -7.7797) knots 0 0 0 1 1 1
  spline S85 degree 2 poles (4.3056, -7.7797) (4.3056, -8.2767) (4.5655, -8.5007) knots 0 0 0 1 1 1
  spline S86 degree 2 poles (4.5655, -8.5007) (4.8255, -8.7246) (5.3813, -8.7246) knots 0 0 0 1 1 1
  line L94 (5.3813, -8.7246) -> (8.3012, -8.7246)
  line L95 (8.3012, -8.7246) -> (8.3012, -9.735)
  spline S87 degree 2 poles (4.8484, -13.7274) (4.201, -13.7274) (3.8282, -13.2614) knots 0 0 0 1 1 1
  spline S88 degree 2 poles (3.8282, -13.2614) (3.4555, -12.7955) (3.4555, -11.965) knots 0 0 0 1 1 1
  spline S89 degree 2 poles (3.4555, -11.965) (3.4555, -11.1998) (3.7432, -10.6113) knots 0 0 0 1 1 1
  line L96 (3.7432, -10.6113) -> (4.6849, -10.6113)
  spline S90 degree 2 poles (4.6849, -10.6113) (4.4691, -11.0952) (4.3808, -11.4304) knots 0 0 0 1 1 1
  spline S91 degree 2 poles (4.3808, -11.4304) (4.2925, -11.7655) (4.2925, -12.0434) knots 0 0 0 1 1 1
  spline S92 degree 2 poles (4.2925, -12.0434) (4.2925, -12.377) (4.42, -12.5552) knots 0 0 0 1 1 1
  spline S93 degree 2 poles (4.42, -12.5552) (4.5476, -12.7334) (4.7993, -12.7334) knots 0 0 0 1 1 1
  spline S94 degree 2 poles (4.7993, -12.7334) (4.9399, -12.7334) (5.0495, -12.6549) knots 0 0 0 1 1 1
  spline S95 degree 2 poles (5.0495, -12.6549) (5.159, -12.5764) (5.2604, -12.4244) knots 0 0 0 1 1 1
  spline S96 degree 2 poles (5.2604, -12.4244) (5.3617, -12.2723) (5.5841, -11.8047) knots 0 0 0 1 1 1
  spline S97 degree 2 poles (5.5841, -11.8047) (5.7901, -11.3666) (5.9797, -11.1475) knots 0 0 0 1 1 1
  spline S98 degree 2 poles (5.9797, -11.1475) (6.1694, -10.9285) (6.4211, -10.7977) knots 0 0 0 1 1 1
  spline S99 degree 2 poles (6.4211, -10.7977) (6.6729, -10.6669) (7.0097, -10.6669) knots 0 0 0 1 1 1
  spline S100 degree 2 poles (7.0097, -10.6669) (7.644, -10.6669) (8.007, -11.0968) knots 0 0 0 1 1 1
  spline S101 degree 2 poles (8.007, -11.0968) (8.3699, -11.5268) (8.3699, -12.2854) knots 0 0 0 1 1 1
  spline S102 degree 2 poles (8.3699, -12.2854) (8.3699, -12.6582) (8.2816, -12.9966) knots 0 0 0 1 1 1
  spline S103 degree 2 poles (8.2816, -12.9966) (8.1933, -13.335) (8.0331, -13.7045) knots 0 0 0 1 1 1
  line L97 (8.0331, -13.7045) -> (7.2451, -13.3775)
  spline S104 degree 2 poles (7.2451, -13.3775) (7.4021, -12.9949) (7.4642, -12.7448) knots 0 0 0 1 1 1
  spline S105 degree 2 poles (7.4642, -12.7448) (7.5263, -12.4947) (7.5263, -12.2527) knots 0 0 0 1 1 1
  spline S106 degree 2 poles (7.5263, -12.2527) (7.5263, -11.965) (7.3922, -11.8113) knots 0 0 0 1 1 1
  spline S107 degree 2 poles (7.3922, -11.8113) (7.2582, -11.6576) (7.0424, -11.6576) knots 0 0 0 1 1 1
  spline S108 degree 2 poles (7.0424, -11.6576) (6.9083, -11.6576) (6.8086, -11.7197) knots 0 0 0 1 1 1
  spline S109 degree 2 poles (6.8086, -11.7197) (6.7089, -11.7819) (6.6157, -11.9176) knots 0 0 0 1 1 1
  spline S110 degree 2 poles (6.6157, -11.9176) (6.5225, -12.0532) (6.2805, -12.5601) knots 0 0 0 1 1 1
  spline S111 degree 2 poles (6.2805, -12.5601) (5.9601, -13.2304) (5.638, -13.4789) knots 0 0 0 1 1 1
  spline S112 degree 2 poles (5.638, -13.4789) (5.316, -13.7274) (4.8484, -13.7274) knots 0 0 0 1 1 1
  line L98 (8.3012, -14.5939) -> (8.3012, -16.0816)
  spline S113 degree 2 poles (8.3012, -16.0816) (8.3012, -17.0985) (8.0119, -17.5579) knots 0 0 0 1 1 1
  spline S114 degree 2 poles (8.0119, -17.5579) (7.7225, -18.0173) (7.0914, -18.0173) knots 0 0 0 1 1 1
  spline S115 degree 2 poles (7.0914, -18.0173) (6.6631, -18.0173) (6.3884, -17.8162) knots 0 0 0 1 1 1
  spline S116 degree 2 poles (6.3884, -17.8162) (6.1138, -17.6151) (6.0582, -17.2816) knots 0 0 0 1 1 1
  line L99 (6.0582, -17.2816) -> (6.0255, -17.2816)
  spline S117 degree 2 poles (6.0255, -17.2816) (5.9241, -17.7361) (5.6462, -17.9372) knots 0 0 0 1 1 1
  spline S118 degree 2 poles (5.6462, -17.9372) (5.3683, -18.1383) (4.9072, -18.1383) knots 0 0 0 1 1 1
  spline S119 degree 2 poles (4.9072, -18.1383) (4.2533, -18.1383) (3.8871, -17.6658) knots 0 0 0 1 1 1
  spline S120 degree 2 poles (3.8871, -17.6658) (3.5209, -17.1933) (3.5209, -16.3824) knots 0 0 0 1 1 1
  line L100 (3.5209, -16.3824) -> (3.5209, -14.5939)
  line L101 (3.5209, -14.5939) -> (8.3012, -14.5939)
  line L102 (6.408, -15.6075) -> (6.408, -16.196)
  spline S121 degree 2 poles (6.408, -16.196) (6.408, -16.608) (6.5356, -16.7928) knots 0 0 0 1 1 1
  spline S122 degree 2 poles (6.5356, -16.7928) (6.6631, -16.9775) (6.9574, -16.9775) knots 0 0 0 1 1 1
  spline S123 degree 2 poles (6.9574, -16.9775) (7.232, -16.9775) (7.3514, -16.7764) knots 0 0 0 1 1 1
  spline S124 degree 2 poles (7.3514, -16.7764) (7.4707, -16.5753) (7.4707, -16.1404) knots 0 0 0 1 1 1
  line L103 (7.4707, -16.1404) -> (7.4707, -15.6075)
  line L104 (7.4707, -15.6075) -> (6.408, -15.6075)
  line L105 (5.6037, -15.6075) -> (4.3579, -15.6075)
  line L106 (4.3579, -15.6075) -> (4.3579, -16.268)
  spline S125 degree 2 poles (4.3579, -16.268) (4.3579, -16.6865) (4.5181, -16.8859) knots 0 0 0 1 1 1
  spline S126 degree 2 poles (4.5181, -16.8859) (4.6783, -17.0854) (5.0086, -17.0854) knots 0 0 0 1 1 1
  spline S127 degree 2 poles (5.0086, -17.0854) (5.6037, -17.0854) (5.6037, -16.2353) knots 0 0 0 1 1 1
  line L107 (5.6037, -16.2353) -> (5.6037, -15.6075)
  spline S128 degree 2 poles (54.9322, -6.3732) (54.9293, -5.1928) (55.5997, -4.5633) knots 0 0 0 1 1 1
  spline S129 degree 2 poles (55.5997, -4.5633) (56.2701, -3.9339) (57.5387, -3.9308) knots 0 0 0 1 1 1
  line L108 (57.5387, -3.9308) -> (58.8924, -3.9274)
  line L109 (58.8924, -3.9274) -> (58.9042, -8.7078)
  line L110 (58.9042, -8.7078) -> (57.4034, -8.7115)
  spline S130 degree 2 poles (57.4034, -8.7115) (56.2328, -8.7144) (55.5839, -8.098) knots 0 0 0 1 1 1
  spline S131 degree 2 poles (55.5839, -8.098) (54.935, -7.4816) (54.9322, -6.3732) knots 0 0 0 1 1 1
  spline S132 degree 2 poles (55.985, -6.3444) (55.9888, -7.8845) (57.349, -7.8811) knots 0 0 0 1 1 1
  line L111 (57.349, -7.8811) -> (57.8885, -7.8798)
  line L112 (57.8885, -7.8798) -> (57.8808, -4.767)
  line L113 (57.8808, -4.767) -> (57.446, -4.768)
  spline S133 degree 2 poles (57.446, -4.768) (55.9811, -4.7717) (55.985, -6.3444) knots 0 0 0 1 1 1
  line L114 (52.0004, -6.8513) -> (52.8636, -6.8491)
  line L115 (52.8636, -6.8491) -> (52.8564, -3.9423)
  line L116 (52.8564, -3.9423) -> (53.8537, -3.9399)
  line L117 (53.8537, -3.9399) -> (53.8609, -6.8467)
  line L118 (53.8609, -6.8467) -> (54.4102, -6.8453)
  line L119 (54.4102, -6.8453) -> (54.4114, -7.326)
  line L120 (54.4114, -7.326) -> (53.8628, -7.5954)
  line L121 (53.8628, -7.5954) -> (53.8634, -7.8636)
  spline S134 degree 2 poles (53.8634, -7.8636) (53.865, -8.4881) (53.5583, -8.7766) knots 0 0 0 1 1 1
  spline S135 degree 2 poles (53.5583, -8.7766) (53.2517, -9.0651) (52.5749, -9.0668) knots 0 0 0 1 1 1
  spline S136 degree 2 poles (52.5749, -9.0668) (52.0582, -9.068) (51.6557, -8.9154) knots 0 0 0 1 1 1
  line L122 (51.6557, -8.9154) -> (51.9089, -8.1823)
  spline S137 degree 2 poles (51.9089, -8.1823) (52.21, -8.2764) (52.465, -8.2757) knots 0 0 0 1 1 1
  spline S138 degree 2 poles (52.465, -8.2757) (52.6775, -8.2752) (52.772, -8.1491) knots 0 0 0 1 1 1
  spline S139 degree 2 poles (52.772, -8.1491) (52.8665, -8.023) (52.8661, -7.8268) knots 0 0 0 1 1 1
  line L123 (52.8661, -7.8268) -> (52.8655, -7.5979)
  line L124 (52.8655, -7.5979) -> (52.0023, -7.6001)
  line L125 (52.0023, -7.6001) -> (52.0004, -6.8513)
  spline S140 degree 2 poles (49.8828, -4.6789) (49.6212, -4.6795) (49.2553, -4.7949) knots 0 0 0 1 1 1
  line L126 (49.2553, -4.7949) -> (49.2534, -4.0526)
  spline S141 degree 2 poles (49.2534, -4.0526) (49.6258, -3.8849) (50.1686, -3.8836) knots 0 0 0 1 1 1
  spline S142 degree 2 poles (50.1686, -3.8836) (50.7669, -3.8821) (51.0407, -4.1839) knots 0 0 0 1 1 1
  spline S143 degree 2 poles (51.0407, -4.1839) (51.3145, -4.4857) (51.316, -5.0906) knots 0 0 0 1 1 1
  line L127 (51.316, -5.0906) -> (51.3203, -6.853)
  line L128 (51.3203, -6.853) -> (51.7977, -6.8518)
  line L129 (51.7977, -6.8518) -> (51.7987, -7.2736)
  line L130 (51.7987, -7.2736) -> (51.2503, -7.6085)
  line L131 (51.2503, -7.6085) -> (50.9644, -8.3808)
  line L132 (50.9644, -8.3808) -> (50.3268, -8.3824)
  line L133 (50.3268, -8.3824) -> (50.3249, -7.6042)
  line L134 (50.3249, -7.6042) -> (49.3015, -7.6067)
  line L135 (49.3015, -7.6067) -> (49.2996, -6.858)
  line L136 (49.2996, -6.858) -> (50.323, -6.8554)
  line L137 (50.323, -6.8554) -> (50.3187, -5.093)
  spline S144 degree 2 poles (50.3187, -5.093) (50.3182, -4.8805) (50.1986, -4.7794) knots 0 0 0 1 1 1
  spline S145 degree 2 poles (50.1986, -4.7794) (50.079, -4.6784) (49.8828, -4.6789) knots 0 0 0 1 1 1
  line L138 (43.9497, -6.6227) -> (43.6227, -6.6235)
  spline S146 degree 2 poles (43.6227, -6.6235) (43.1421, -6.6247) (42.9136, -6.7855) knots 0 0 0 1 1 1
  spline S147 degree 2 poles (42.9136, -6.7855) (42.6851, -6.9463) (42.686, -7.2896) knots 0 0 0 1 1 1
  spline S148 degree 2 poles (42.686, -7.2896) (42.6868, -7.6297) (42.9209, -7.7729) knots 0 0 0 1 1 1
  spline S149 degree 2 poles (42.9209, -7.7729) (43.1551, -7.9162) (43.6455, -7.915) knots 0 0 0 1 1 1
  line L139 (43.6455, -7.915) -> (43.9529, -7.9143)
  line L140 (43.9529, -7.9143) -> (43.9497, -6.6227)
  line L141 (43.9477, -5.7987) -> (43.9431, -3.9644)
  line L142 (43.9431, -3.9644) -> (44.9567, -3.9619)
  line L143 (44.9567, -3.9619) -> (44.9686, -8.7423)
  line L144 (44.9686, -8.7423) -> (43.5757, -8.7457)
  spline S150 degree 2 poles (43.5757, -8.7457) (42.6013, -8.7481) (42.1328, -8.3945) knots 0 0 0 1 1 1
  spline S151 degree 2 poles (42.1328, -8.3945) (41.6644, -8.0409) (41.6626, -7.3183) knots 0 0 0 1 1 1
  spline S152 degree 2 poles (41.6626, -7.3183) (41.6615, -6.8965) (41.8929, -6.5673) knots 0 0 0 1 1 1
  spline S153 degree 2 poles (41.8929, -6.5673) (42.1242, -6.2381) (42.5488, -6.0507) knots 0 0 0 1 1 1
  spline S154 degree 2 poles (42.5488, -6.0507) (41.4658, -4.4414) (41.1377, -3.9714) knots 0 0 0 1 1 1
  line L145 (41.1377, -3.9714) -> (42.2625, -3.9686)
  line L146 (42.2625, -3.9686) -> (43.4082, -5.8001)
  line L147 (43.4082, -5.8001) -> (43.9477, -5.7987)
  spline S155 degree 2 poles (38.0668, -5.0645) (38.0654, -4.5021) (38.4554, -4.2069) knots 0 0 0 1 1 1
  spline S156 degree 2 poles (38.4554, -4.2069) (38.8454, -3.9116) (39.6236, -3.9097) knots 0 0 0 1 1 1
  spline S157 degree 2 poles (39.6236, -3.9097) (40.0225, -3.9087) (40.3039, -3.962) knots 0 0 0 1 1 1
  spline S158 degree 2 poles (40.3039, -3.962) (40.5852, -4.0152) (40.8307, -4.1193) knots 0 0 0 1 1 1
  line L148 (40.8307, -4.1193) -> (40.8327, -4.9432)
  spline S159 degree 2 poles (40.8327, -4.9432) (40.5545, -4.8131) (40.206, -4.7257) knots 0 0 0 1 1 1
  spline S160 degree 2 poles (40.206, -4.7257) (39.8576, -4.6383) (39.5927, -4.6389) knots 0 0 0 1 1 1
  spline S161 degree 2 poles (39.5927, -4.6389) (39.05, -4.6403) (39.0507, -4.9542) knots 0 0 0 1 1 1
  spline S162 degree 2 poles (39.0507, -4.9542) (39.051, -5.0719) (39.1231, -5.1453) knots 0 0 0 1 1 1
  spline S163 degree 2 poles (39.1231, -5.1453) (39.1953, -5.2187) (39.3721, -5.3114) knots 0 0 0 1 1 1
  spline S164 degree 2 poles (39.3721, -5.3114) (39.5489, -5.4042) (39.8434, -5.5277) knots 0 0 0 1 1 1
  spline S165 degree 2 poles (39.8434, -5.5277) (40.2657, -5.7032) (40.4639, -5.8531) knots 0 0 0 1 1 1
  spline S166 degree 2 poles (40.4639, -5.8531) (40.6621, -6.0031) (40.7525, -6.1974) knots 0 0 0 1 1 1
  spline S167 degree 2 poles (40.7525, -6.1974) (40.8429, -6.3917) (40.8436, -6.6762) knots 0 0 0 1 1 1
  spline S168 degree 2 poles (40.8436, -6.6762) (40.8448, -7.1634) (40.4678, -7.4308) knots 0 0 0 1 1 1
  spline S169 degree 2 poles (40.4678, -7.4308) (40.0908, -7.6982) (39.3976, -7.6999) knots 0 0 0 1 1 1
  spline S170 degree 2 poles (39.3976, -7.6999) (38.7371, -7.7016) (38.1119, -7.4154) knots 0 0 0 1 1 1
  line L149 (38.1119, -7.4154) -> (38.4109, -6.6953)
  spline S171 degree 2 poles (38.4109, -6.6953) (38.6858, -6.8123) (38.9247, -6.8869) knots 0 0 0 1 1 1
  spline S172 degree 2 poles (38.9247, -6.8869) (39.1636, -6.9615) (39.4121, -6.9609) knots 0 0 0 1 1 1
  spline S173 degree 2 poles (39.4121, -6.9609) (39.8535, -6.9598) (39.8529, -6.7211) knots 0 0 0 1 1 1
  spline S174 degree 2 poles (39.8529, -6.7211) (39.8526, -6.5871) (39.7101, -6.4893) knots 0 0 0 1 1 1
  spline S175 degree 2 poles (39.7101, -6.4893) (39.5676, -6.3916) (39.0865, -6.1999) knots 0 0 0 1 1 1
  spline S176 degree 2 poles (39.0865, -6.1999) (38.6577, -6.0276) (38.4579, -5.8777) knots 0 0 0 1 1 1
  spline S177 degree 2 poles (38.4579, -5.8777) (38.2581, -5.7278) (38.1628, -5.5319) knots 0 0 0 1 1 1
  spline S178 degree 2 poles (38.1628, -5.5319) (38.0675, -5.3359) (38.0668, -5.0645) knots 0 0 0 1 1 1
  spline S179 degree 2 poles (35.7477, -4.7139) (35.4861, -4.7145) (35.1202, -4.8298) knots 0 0 0 1 1 1
  line L150 (35.1202, -4.8298) -> (35.1183, -4.0876)
  spline S180 degree 2 poles (35.1183, -4.0876) (35.4907, -3.9199) (36.0334, -3.9186) knots 0 0 0 1 1 1
  spline S181 degree 2 poles (36.0334, -3.9186) (36.6318, -3.9171) (36.9056, -4.2189) knots 0 0 0 1 1 1
  spline S182 degree 2 poles (36.9056, -4.2189) (37.1794, -4.5207) (37.1809, -5.1256) knots 0 0 0 1 1 1
  line L151 (37.1809, -5.1256) -> (37.1852, -6.888)
  line L152 (37.1852, -6.888) -> (37.6626, -6.8868)
  line L153 (37.6626, -6.8868) -> (37.6636, -7.3086)
  line L154 (37.6636, -7.3086) -> (37.1152, -7.6434)
  line L155 (37.1152, -7.6434) -> (36.8293, -8.4158)
  line L156 (36.8293, -8.4158) -> (36.1917, -8.4174)
  line L157 (36.1917, -8.4174) -> (36.1898, -7.6392)
  line L158 (36.1898, -7.6392) -> (35.1664, -7.6417)
  line L159 (35.1664, -7.6417) -> (35.1645, -6.893)
  line L160 (35.1645, -6.893) -> (36.1879, -6.8904)
  line L161 (36.1879, -6.8904) -> (36.1836, -5.128)
  spline S183 degree 2 poles (36.1836, -5.128) (36.1831, -4.9155) (36.0635, -4.8144) knots 0 0 0 1 1 1
  spline S184 degree 2 poles (36.0635, -4.8144) (35.9439, -4.7134) (35.7477, -4.7139) knots 0 0 0 1 1 1
  line L162 (81.156, -28.413) -> (81.156, -28.0795)
  spline S185 degree 2 poles (81.156, -28.0795) (81.156, -27.6119) (80.9712, -27.3798) knots 0 0 0 1 1 1
  spline S186 degree 2 poles (80.9712, -27.3798) (80.7865, -27.1476) (80.4334, -27.1476) knots 0 0 0 1 1 1
  spline S187 degree 2 poles (80.4334, -27.1476) (80.077, -27.1476) (79.9069, -27.3421) knots 0 0 0 1 1 1
  spline S188 degree 2 poles (79.9069, -27.3421) (79.7369, -27.5367) (79.7369, -27.952) knots 0 0 0 1 1 1
  line L163 (79.7369, -27.952) -> (79.7369, -28.413)
  line L164 (79.7369, -28.413) -> (81.156, -28.413)
  spline S189 degree 2 poles (80.3974, -26.1242) (81.1691, -26.1242) (81.5778, -26.6065) knots 0 0 0 1 1 1
  spline S190 degree 2 poles (81.5778, -26.6065) (81.9865, -27.0887) (81.9865, -27.9781) knots 0 0 0 1 1 1
  line L165 (81.9865, -27.9781) -> (81.9865, -28.413)
  line L166 (81.9865, -28.413) -> (83.6868, -28.413)
  line L167 (83.6868, -28.413) -> (83.6868, -29.4266)
  line L168 (83.6868, -29.4266) -> (78.9064, -29.4266)
  line L169 (78.9064, -29.4266) -> (78.9064, -27.8996)
  spline S191 degree 2 poles (78.9064, -27.8996) (78.9064, -27.0299) (79.2808, -26.577) knots 0 0 0 1 1 1